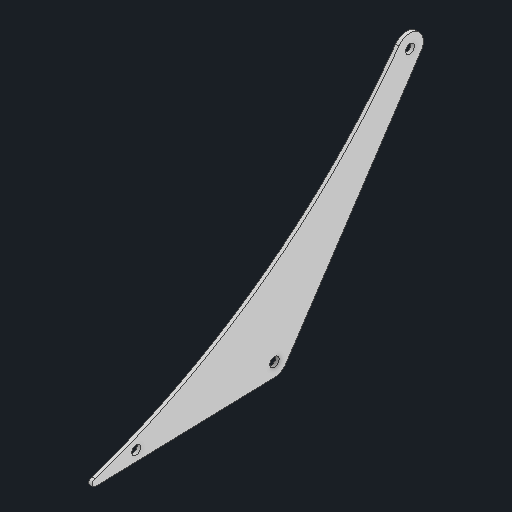
# Autodesk Inventor part: ramp
Saved by Autodesk Inventor 2025 (Build 290162000, 162)
## iProperties
Created: 2024-10-13
Part Number: ramp
Material: Generic
Document SubType Name: Modeling
Designer: Averey Ku
Density: 1 g/cm^3
Appearance: Default
Author: Averey Ku
Autodesk Inventor part; units mm, degrees
ref_plane "YZ Plane" through (0, 0, 0) normal (1, 0, 0) x (0, 1, 0)
ref_plane "XZ Plane" through (0, 0, 0) normal (0, 1, 0) x (-1, 0, 0)
ref_plane "XY Plane" through (0, 0, 0) normal (0, 0, 1) x (1, 0, 0)
sketch "main" plane through (0, 0, 0) normal (0, 0, 1) x (1, 0, 0)
  circle A0 centre (-44.1104, -6.7217) radius 2.1844
  circle A1 centre (51.8207, -70.5484) radius 2.1
  arc A2 (47.9474, -75.5803) -> (55.5576, -65.4144) centre (51.8207, -70.5484) ccw
  arc A3 (-49.5996, 77.7257) -> (-52.7448, 77.3832) centre (-51.1867, 77.6872) ccw
  arc A4 (-50.458, -6.8955) -> (-47.6279, -12.0084) centre (-44.1104, -6.7217) ccw
  line L0 (-52.7736, 77.6438) -> (-50.458, -6.8955)
  line L1 (48.3032, -75.8352) -> (-47.6279, -12.0084)
  arc A5 (-49.5996, 77.7257) -> (55.5576, -65.4144) centre (227.9515, 171.4307) ccw
  circle A6 centre (-47.4837, 58.4542) radius 2.0828
  point P0 (1.1251, 9.7944)
  point P1 (-13.7084, -66.6167)
  point P2 (-7.1584, -6.3825)
  dimension "d5" = 12.7
  dimension "d6" = 4.1656
  measures "d5" diameter of A4
  measures "d6" diameter of A6
sketch "Sketch1" plane through (0, 0, 0) normal (1, 0, 0) x (0, 1, 0)
  circle A0 centre (0, 0) radius 2.1844
  circle A1 centre (95.9311, -63.8268) radius 2.1
  arc A2 (92.0578, -68.8587) -> (99.668, -58.6928) centre (95.9311, -63.8268) ccw
  arc A3 (-5.4892, 84.4473) -> (-8.6344, 84.1049) centre (-7.0763, 84.4089) ccw
  arc A4 (-6.3476, -0.1739) -> (-3.5175, -5.2868) centre (0, 0) ccw
  line L0 (-8.6632, 84.3654) -> (-6.3476, -0.1739)
  line L1 (92.4136, -69.1135) -> (-3.5175, -5.2868)
  arc A5 (-5.4892, 84.4473) -> (99.668, -58.6928) centre (272.0619, 178.1523) ccw
  circle A6 centre (-3.3733, 65.1759) radius 2.0828
  constraints: 1 other
extrude "Extrusion1" add sketch "Sketch1" along normal blind 1.5875
body "Solid1"
